Autodesk Fusion 360 part; units mm, degrees
(part 13 of 14)
  line L9122 (-513.1939, 44.45) -> (-524.1924, 44.45)
  line L9123 (-524.1924, 44.45) -> (-529.6916, 34.925)
  line L9124 (-529.6916, 34.925) -> (-524.1924, 25.4)
  line L9125 (-524.1924, 25.4) -> (-513.1939, 25.4)
  line L9126 (-507.6946, 34.925) -> (-513.1939, 44.45)
  line L9127 (-513.1939, 25.4) -> (-507.6946, 34.925)
  line L9128 (-493.9464, 55.5625) -> (-504.945, 55.5625)
  line L9129 (-504.945, 55.5625) -> (-510.4442, 46.0375)
  line L9130 (-510.4442, 46.0375) -> (-504.945, 36.5125)
  line L9131 (-504.945, 36.5125) -> (-493.9464, 36.5125)
  line L9132 (-488.4472, 46.0375) -> (-493.9464, 55.5625)
  line L9133 (-493.9464, 36.5125) -> (-488.4472, 46.0375)
  line L9134 (-474.699, 66.675) -> (-485.6976, 66.675)
  line L9135 (-485.6976, 66.675) -> (-491.1968, 57.15)
  line L9136 (-491.1968, 57.15) -> (-485.6976, 47.625)
  line L9137 (-485.6976, 47.625) -> (-474.699, 47.625)
  line L9138 (-469.1998, 57.15) -> (-474.699, 66.675)
  line L9139 (-474.699, 47.625) -> (-469.1998, 57.15)
  line L9140 (-455.4516, 77.7875) -> (-466.4501, 77.7875)
  line L9141 (-466.4501, 77.7875) -> (-471.9494, 68.2625)
  line L9142 (-471.9494, 68.2625) -> (-466.4501, 58.7375)
  line L9143 (-466.4501, 58.7375) -> (-455.4516, 58.7375)
  line L9144 (-449.9524, 68.2625) -> (-455.4516, 77.7875)
  line L9145 (-455.4516, 58.7375) -> (-449.9524, 68.2625)
  line L9146 (-436.2042, 88.9) -> (-447.2027, 88.9)
  line L9147 (-447.2027, 88.9) -> (-452.702, 79.375)
  line L9148 (-452.702, 79.375) -> (-447.2027, 69.85)
  line L9149 (-447.2027, 69.85) -> (-436.2042, 69.85)
  line L9150 (-430.7049, 79.375) -> (-436.2042, 88.9)
  line L9151 (-436.2042, 69.85) -> (-430.7049, 79.375)
  line L9152 (-416.9568, 100.0125) -> (-427.9553, 100.0125)
  line L9153 (-427.9553, 100.0125) -> (-433.4546, 90.4875)
  line L9154 (-433.4546, 90.4875) -> (-427.9553, 80.9625)
  line L9155 (-427.9553, 80.9625) -> (-416.9568, 80.9625)
  line L9156 (-411.4575, 90.4875) -> (-416.9568, 100.0125)
  line L9157 (-416.9568, 80.9625) -> (-411.4575, 90.4875)
  line L9158 (-397.7094, 111.125) -> (-408.7079, 111.125)
  line L9159 (-408.7079, 111.125) -> (-414.2072, 101.6)
  line L9160 (-414.2072, 101.6) -> (-408.7079, 92.075)
  line L9161 (-408.7079, 92.075) -> (-397.7094, 92.075)
  line L9162 (-392.2101, 101.6) -> (-397.7094, 111.125)
  line L9163 (-397.7094, 92.075) -> (-392.2101, 101.6)
  line L9164 (-378.462, 122.2375) -> (-389.4605, 122.2375)
  line L9165 (-389.4605, 122.2375) -> (-394.9597, 112.7125)
  line L9166 (-394.9597, 112.7125) -> (-389.4605, 103.1875)
  line L9167 (-389.4605, 103.1875) -> (-378.462, 103.1875)
  line L9168 (-372.9627, 112.7125) -> (-378.462, 122.2375)
  line L9169 (-378.462, 103.1875) -> (-372.9627, 112.7125)
  line L9170 (-359.2145, 133.35) -> (-370.2131, 133.35)
  line L9171 (-370.2131, 133.35) -> (-375.7123, 123.825)
  line L9172 (-375.7123, 123.825) -> (-370.2131, 114.3)
  line L9173 (-370.2131, 114.3) -> (-359.2145, 114.3)
  line L9174 (-353.7153, 123.825) -> (-359.2145, 133.35)
  line L9175 (-359.2145, 114.3) -> (-353.7153, 123.825)
  line L9176 (-339.9671, 144.4625) -> (-350.9657, 144.4625)
  line L9177 (-350.9657, 144.4625) -> (-356.4649, 134.9375)
  line L9178 (-356.4649, 134.9375) -> (-350.9657, 125.4125)
  line L9179 (-350.9657, 125.4125) -> (-339.9671, 125.4125)
  line L9180 (-334.4679, 134.9375) -> (-339.9671, 144.4625)
  line L9181 (-339.9671, 125.4125) -> (-334.4679, 134.9375)
  line L9182 (-320.7197, 155.575) -> (-331.7182, 155.575)
  line L9183 (-331.7182, 155.575) -> (-337.2175, 146.05)
  line L9184 (-337.2175, 146.05) -> (-331.7182, 136.525)
  line L9185 (-331.7182, 136.525) -> (-320.7197, 136.525)
  line L9186 (-315.2205, 146.05) -> (-320.7197, 155.575)
  line L9187 (-320.7197, 136.525) -> (-315.2205, 146.05)
  line L9188 (-301.4723, 166.6875) -> (-312.4708, 166.6875)
  line L9189 (-312.4708, 166.6875) -> (-317.9701, 157.1625)
  line L9190 (-317.9701, 157.1625) -> (-312.4708, 147.6375)
  line L9191 (-312.4708, 147.6375) -> (-301.4723, 147.6375)
  line L9192 (-295.973, 157.1625) -> (-301.4723, 166.6875)
  line L9193 (-301.4723, 147.6375) -> (-295.973, 157.1625)
  line L9194 (-282.2249, 177.8) -> (-293.2234, 177.8)
  line L9195 (-293.2234, 177.8) -> (-298.7227, 168.275)
  line L9196 (-298.7227, 168.275) -> (-293.2234, 158.75)
  line L9197 (-293.2234, 158.75) -> (-282.2249, 158.75)
  line L9198 (-276.7256, 168.275) -> (-282.2249, 177.8)
  line L9199 (-282.2249, 158.75) -> (-276.7256, 168.275)
  line L9200 (-262.9775, 188.9125) -> (-273.976, 188.9125)
  line L9201 (-273.976, 188.9125) -> (-279.4753, 179.3875)
  line L9202 (-279.4753, 179.3875) -> (-273.976, 169.8625)
  line L9203 (-273.976, 169.8625) -> (-262.9775, 169.8625)
  line L9204 (-257.4782, 179.3875) -> (-262.9775, 188.9125)
  line L9205 (-262.9775, 169.8625) -> (-257.4782, 179.3875)
  line L9206 (-243.7301, 200.025) -> (-254.7286, 200.025)
  line L9207 (-254.7286, 200.025) -> (-260.2278, 190.5)
  line L9208 (-260.2278, 190.5) -> (-254.7286, 180.975)
  line L9209 (-254.7286, 180.975) -> (-243.7301, 180.975)
  line L9210 (-238.2308, 190.5) -> (-243.7301, 200.025)
  line L9211 (-243.7301, 180.975) -> (-238.2308, 190.5)
  line L9212 (-224.4826, 211.1375) -> (-235.4812, 211.1375)
  line L9213 (-235.4812, 211.1375) -> (-240.9804, 201.6125)
  line L9214 (-240.9804, 201.6125) -> (-235.4812, 192.0875)
  line L9215 (-235.4812, 192.0875) -> (-224.4826, 192.0875)
  line L9216 (-218.9834, 201.6125) -> (-224.4826, 211.1375)
  line L9217 (-224.4826, 192.0875) -> (-218.9834, 201.6125)
  line L9218 (-205.2352, 222.25) -> (-216.2337, 222.25)
  line L9219 (-216.2337, 222.25) -> (-221.733, 212.725)
  line L9220 (-221.733, 212.725) -> (-216.2337, 203.2)
  line L9221 (-216.2337, 203.2) -> (-205.2352, 203.2)
  line L9222 (-199.736, 212.725) -> (-205.2352, 222.25)
  line L9223 (-205.2352, 203.2) -> (-199.736, 212.725)
  line L9224 (-185.9878, 233.3625) -> (-196.9863, 233.3625)
  line L9225 (-196.9863, 233.3625) -> (-202.4856, 223.8375)
  line L9226 (-202.4856, 223.8375) -> (-196.9863, 214.3125)
  line L9227 (-196.9863, 214.3125) -> (-185.9878, 214.3125)
  line L9228 (-180.4886, 223.8375) -> (-185.9878, 233.3625)
  line L9229 (-185.9878, 214.3125) -> (-180.4886, 223.8375)
  line L9230 (-166.7404, 244.475) -> (-177.7389, 244.475)
  line L9231 (-177.7389, 244.475) -> (-183.2382, 234.95)
  line L9232 (-183.2382, 234.95) -> (-177.7389, 225.425)
  line L9233 (-177.7389, 225.425) -> (-166.7404, 225.425)
  line L9234 (-161.2411, 234.95) -> (-166.7404, 244.475)
  line L9235 (-166.7404, 225.425) -> (-161.2411, 234.95)
  line L9236 (-147.493, 255.5875) -> (-158.4915, 255.5875)
  line L9237 (-158.4915, 255.5875) -> (-163.9908, 246.0625)
  line L9238 (-163.9908, 246.0625) -> (-158.4915, 236.5375)
  line L9239 (-158.4915, 236.5375) -> (-147.493, 236.5375)
  line L9240 (-141.9937, 246.0625) -> (-147.493, 255.5875)
  line L9241 (-147.493, 236.5375) -> (-141.9937, 246.0625)
  line L9242 (-128.2456, 266.7) -> (-139.2441, 266.7)
  line L9243 (-139.2441, 266.7) -> (-144.7434, 257.175)
  line L9244 (-144.7434, 257.175) -> (-139.2441, 247.65)
  line L9245 (-139.2441, 247.65) -> (-128.2456, 247.65)
  line L9246 (-122.7463, 257.175) -> (-128.2456, 266.7)
  line L9247 (-128.2456, 247.65) -> (-122.7463, 257.175)
  line L9248 (-108.9982, 277.8125) -> (-119.9967, 277.8125)
  line L9249 (-119.9967, 277.8125) -> (-125.4959, 268.2875)
  line L9250 (-125.4959, 268.2875) -> (-119.9967, 258.7625)
  line L9251 (-119.9967, 258.7625) -> (-108.9982, 258.7625)
  line L9252 (-103.4989, 268.2875) -> (-108.9982, 277.8125)
  line L9253 (-108.9982, 258.7625) -> (-103.4989, 268.2875)
  line L9254 (-89.7507, 288.925) -> (-100.7493, 288.925)
  line L9255 (-100.7493, 288.925) -> (-106.2485, 279.4)
  line L9256 (-106.2485, 279.4) -> (-100.7493, 269.875)
  line L9257 (-100.7493, 269.875) -> (-89.7507, 269.875)
  line L9258 (-84.2515, 279.4) -> (-89.7507, 288.925)
  line L9259 (-89.7507, 269.875) -> (-84.2515, 279.4)
  line L9260 (-70.5033, 300.0375) -> (-81.5018, 300.0375)
  line L9261 (-81.5018, 300.0375) -> (-87.0011, 290.5125)
  line L9262 (-87.0011, 290.5125) -> (-81.5018, 280.9875)
  line L9263 (-81.5018, 280.9875) -> (-70.5033, 280.9875)
  line L9264 (-65.0041, 290.5125) -> (-70.5033, 300.0375)
  line L9265 (-70.5033, 280.9875) -> (-65.0041, 290.5125)
  line L9266 (-51.2559, 311.15) -> (-62.2544, 311.15)
  line L9267 (-62.2544, 311.15) -> (-67.7537, 301.625)
  line L9268 (-67.7537, 301.625) -> (-62.2544, 292.1)
  line L9269 (-62.2544, 292.1) -> (-51.2559, 292.1)
  line L9270 (-45.7566, 301.625) -> (-51.2559, 311.15)
  line L9271 (-51.2559, 292.1) -> (-45.7566, 301.625)
  line L9272 (-32.0085, 322.2625) -> (-43.007, 322.2625)
  line L9273 (-43.007, 322.2625) -> (-48.5063, 312.7375)
  line L9274 (-48.5063, 312.7375) -> (-43.007, 303.2125)
  line L9275 (-43.007, 303.2125) -> (-32.0085, 303.2125)
  line L9276 (-26.5092, 312.7375) -> (-32.0085, 322.2625)
  line L9277 (-32.0085, 303.2125) -> (-26.5092, 312.7375)
  line L9278 (-12.7611, 333.375) -> (-23.7596, 333.375)
  line L9279 (-23.7596, 333.375) -> (-29.2589, 323.85)
  line L9280 (-29.2589, 323.85) -> (-23.7596, 314.325)
  line L9281 (-23.7596, 314.325) -> (-12.7611, 314.325)
  line L9282 (-7.2618, 323.85) -> (-12.7611, 333.375)
  line L9283 (-12.7611, 314.325) -> (-7.2618, 323.85)
  line L9284 (6.4863, 344.4875) -> (-4.5122, 344.4875)
  line L9285 (-4.5122, 344.4875) -> (-10.0114, 334.9625)
  line L9286 (-10.0114, 334.9625) -> (-4.5122, 325.4375)
  line L9287 (-4.5122, 325.4375) -> (6.4863, 325.4375)
  line L9288 (11.9856, 334.9625) -> (6.4863, 344.4875)
  line L9289 (6.4863, 325.4375) -> (11.9856, 334.9625)
  line L9290 (25.7337, 355.6) -> (14.7352, 355.6)
  line L9291 (14.7352, 355.6) -> (9.236, 346.075)
  line L9292 (9.236, 346.075) -> (14.7352, 336.55)
  line L9293 (14.7352, 336.55) -> (25.7337, 336.55)
  line L9294 (31.233, 346.075) -> (25.7337, 355.6)
  line L9295 (25.7337, 336.55) -> (31.233, 346.075)
  line L9296 (44.9812, 366.7125) -> (33.9826, 366.7125)
  line L9297 (33.9826, 366.7125) -> (28.4834, 357.1875)
  line L9298 (28.4834, 357.1875) -> (33.9826, 347.6625)
  line L9299 (33.9826, 347.6625) -> (44.9812, 347.6625)
  line L9300 (50.4804, 357.1875) -> (44.9812, 366.7125)
  line L9301 (44.9812, 347.6625) -> (50.4804, 357.1875)
  line L9302 (64.2286, 377.825) -> (53.2301, 377.825)
  line L9303 (53.2301, 377.825) -> (47.7308, 368.3)
  line L9304 (47.7308, 368.3) -> (53.2301, 358.775)
  line L9305 (53.2301, 358.775) -> (64.2286, 358.775)
  line L9306 (69.7278, 368.3) -> (64.2286, 377.825)
  line L9307 (64.2286, 358.775) -> (69.7278, 368.3)
  line L9308 (83.476, 388.9375) -> (72.4775, 388.9375)
  line L9309 (72.4775, 388.9375) -> (66.9782, 379.4125)
  line L9310 (66.9782, 379.4125) -> (72.4775, 369.8875)
  line L9311 (72.4775, 369.8875) -> (83.476, 369.8875)
  line L9312 (88.9753, 379.4125) -> (83.476, 388.9375)
  line L9313 (83.476, 369.8875) -> (88.9753, 379.4125)
  line L9314 (102.7234, 400.05) -> (91.7249, 400.05)
  line L9315 (91.7249, 400.05) -> (86.2256, 390.525)
  line L9316 (86.2256, 390.525) -> (91.7249, 381)
  line L9317 (91.7249, 381) -> (102.7234, 381)
  line L9318 (108.2227, 390.525) -> (102.7234, 400.05)
  line L9319 (102.7234, 381) -> (108.2227, 390.525)
  line L9320 (121.9708, 411.1625) -> (110.9723, 411.1625)
  line L9321 (110.9723, 411.1625) -> (105.473, 401.6375)
  line L9322 (105.473, 401.6375) -> (110.9723, 392.1125)
  line L9323 (110.9723, 392.1125) -> (121.9708, 392.1125)
  line L9324 (127.4701, 401.6375) -> (121.9708, 411.1625)
  line L9325 (121.9708, 392.1125) -> (127.4701, 401.6375)
  line L9326 (141.2182, 422.275) -> (130.2197, 422.275)
  line L9327 (130.2197, 422.275) -> (124.7205, 412.75)
  line L9328 (124.7205, 412.75) -> (130.2197, 403.225)
  line L9329 (130.2197, 403.225) -> (141.2182, 403.225)
  line L9330 (146.7175, 412.75) -> (141.2182, 422.275)
  line L9331 (141.2182, 403.225) -> (146.7175, 412.75)
  line L9332 (160.4657, 433.3875) -> (149.4671, 433.3875)
  line L9333 (149.4671, 433.3875) -> (143.9679, 423.8625)
  line L9334 (143.9679, 423.8625) -> (149.4671, 414.3375)
  line L9335 (149.4671, 414.3375) -> (160.4657, 414.3375)
  line L9336 (165.9649, 423.8625) -> (160.4657, 433.3875)
  line L9337 (160.4657, 414.3375) -> (165.9649, 423.8625)
  line L9338 (179.7131, 444.5) -> (168.7145, 444.5)
  line L9339 (168.7145, 444.5) -> (163.2153, 434.975)
  line L9340 (163.2153, 434.975) -> (168.7145, 425.45)
  line L9341 (168.7145, 425.45) -> (179.7131, 425.45)
  line L9342 (185.2123, 434.975) -> (179.7131, 444.5)
  line L9343 (179.7131, 425.45) -> (185.2123, 434.975)
  line L9344 (198.9605, 455.6125) -> (187.962, 455.6125)
  line L9345 (187.962, 455.6125) -> (182.4627, 446.0875)
  line L9346 (182.4627, 446.0875) -> (187.962, 436.5625)
  line L9347 (187.962, 436.5625) -> (198.9605, 436.5625)
  line L9348 (204.4597, 446.0875) -> (198.9605, 455.6125)
  line L9349 (198.9605, 436.5625) -> (204.4597, 446.0875)
  line L9350 (218.2079, 466.725) -> (207.2094, 466.725)
  line L9351 (207.2094, 466.725) -> (201.7101, 457.2)
  line L9352 (201.7101, 457.2) -> (207.2094, 447.675)
  line L9353 (207.2094, 447.675) -> (218.2079, 447.675)
  line L9354 (223.7072, 457.2) -> (218.2079, 466.725)
  line L9355 (218.2079, 447.675) -> (223.7072, 457.2)
  line L9356 (237.4553, 477.8375) -> (226.4568, 477.8375)
  line L9357 (226.4568, 477.8375) -> (220.9575, 468.3125)
  line L9358 (220.9575, 468.3125) -> (226.4568, 458.7875)
  line L9359 (226.4568, 458.7875) -> (237.4553, 458.7875)
  line L9360 (242.9546, 468.3125) -> (237.4553, 477.8375)
  line L9361 (237.4553, 458.7875) -> (242.9546, 468.3125)
  line L9362 (256.7027, 488.95) -> (245.7042, 488.95)
  line L9363 (245.7042, 488.95) -> (240.2049, 479.425)
  line L9364 (240.2049, 479.425) -> (245.7042, 469.9)
  line L9365 (245.7042, 469.9) -> (256.7027, 469.9)
  line L9366 (262.202, 479.425) -> (256.7027, 488.95)
  line L9367 (256.7027, 469.9) -> (262.202, 479.425)
  line L9368 (275.9501, 500.0625) -> (264.9516, 500.0625)
  line L9369 (264.9516, 500.0625) -> (259.4524, 490.5375)
  line L9370 (259.4524, 490.5375) -> (264.9516, 481.0125)
  line L9371 (264.9516, 481.0125) -> (275.9501, 481.0125)
  line L9372 (281.4494, 490.5375) -> (275.9501, 500.0625)
  line L9373 (275.9501, 481.0125) -> (281.4494, 490.5375)
  line L9374 (-878.8947, -144.4625) -> (-889.8933, -144.4625)
  line L9375 (-889.8933, -144.4625) -> (-895.3925, -153.9875)
  line L9376 (-895.3925, -153.9875) -> (-889.8933, -163.5125)
  line L9377 (-889.8933, -163.5125) -> (-878.8947, -163.5125)
  line L9378 (-873.3955, -153.9875) -> (-878.8947, -144.4625)
  line L9379 (-878.8947, -163.5125) -> (-873.3955, -153.9875)
  line L9380 (-859.6473, -133.35) -> (-870.6458, -133.35)
  line L9381 (-870.6458, -133.35) -> (-876.1451, -142.875)
  line L9382 (-876.1451, -142.875) -> (-870.6458, -152.4)
  line L9383 (-870.6458, -152.4) -> (-859.6473, -152.4)
  line L9384 (-854.1481, -142.875) -> (-859.6473, -133.35)
  line L9385 (-859.6473, -152.4) -> (-854.1481, -142.875)
  line L9386 (-840.3999, -122.2375) -> (-851.3984, -122.2375)
  line L9387 (-851.3984, -122.2375) -> (-856.8977, -131.7625)
  line L9388 (-856.8977, -131.7625) -> (-851.3984, -141.2875)
  line L9389 (-851.3984, -141.2875) -> (-840.3999, -141.2875)
  line L9390 (-834.9006, -131.7625) -> (-840.3999, -122.2375)
  line L9391 (-840.3999, -141.2875) -> (-834.9006, -131.7625)
  line L9392 (-821.1525, -111.125) -> (-832.151, -111.125)
  line L9393 (-832.151, -111.125) -> (-837.6503, -120.65)
  line L9394 (-837.6503, -120.65) -> (-832.151, -130.175)
  line L9395 (-832.151, -130.175) -> (-821.1525, -130.175)
  line L9396 (-815.6532, -120.65) -> (-821.1525, -111.125)
  line L9397 (-821.1525, -130.175) -> (-815.6532, -120.65)
  line L9398 (-801.9051, -100.0125) -> (-812.9036, -100.0125)
  line L9399 (-812.9036, -100.0125) -> (-818.4029, -109.5375)
  line L9400 (-818.4029, -109.5375) -> (-812.9036, -119.0625)
  line L9401 (-812.9036, -119.0625) -> (-801.9051, -119.0625)
  line L9402 (-796.4058, -109.5375) -> (-801.9051, -100.0125)
  line L9403 (-801.9051, -119.0625) -> (-796.4058, -109.5375)
  line L9404 (-782.6577, -88.9) -> (-793.6562, -88.9)
  line L9405 (-793.6562, -88.9) -> (-799.1554, -98.425)
  line L9406 (-799.1554, -98.425) -> (-793.6562, -107.95)
  line L9407 (-793.6562, -107.95) -> (-782.6577, -107.95)
  line L9408 (-777.1584, -98.425) -> (-782.6577, -88.9)
  line L9409 (-782.6577, -107.95) -> (-777.1584, -98.425)
  line L9410 (-763.4102, -77.7875) -> (-774.4088, -77.7875)
  line L9411 (-774.4088, -77.7875) -> (-779.908, -87.3125)
  line L9412 (-779.908, -87.3125) -> (-774.4088, -96.8375)
  line L9413 (-774.4088, -96.8375) -> (-763.4102, -96.8375)
  line L9414 (-757.911, -87.3125) -> (-763.4102, -77.7875)
  line L9415 (-763.4102, -96.8375) -> (-757.911, -87.3125)
  line L9416 (-744.1628, -66.675) -> (-755.1614, -66.675)
  line L9417 (-755.1614, -66.675) -> (-760.6606, -76.2)
  line L9418 (-760.6606, -76.2) -> (-755.1614, -85.725)
  line L9419 (-755.1614, -85.725) -> (-744.1628, -85.725)
  line L9420 (-738.6636, -76.2) -> (-744.1628, -66.675)
  line L9421 (-744.1628, -85.725) -> (-738.6636, -76.2)
  line L9422 (-724.9154, -55.5625) -> (-735.9139, -55.5625)
  line L9423 (-735.9139, -55.5625) -> (-741.4132, -65.0875)
  line L9424 (-741.4132, -65.0875) -> (-735.9139, -74.6125)
  line L9425 (-735.9139, -74.6125) -> (-724.9154, -74.6125)
  line L9426 (-719.4162, -65.0875) -> (-724.9154, -55.5625)
  line L9427 (-724.9154, -74.6125) -> (-719.4162, -65.0875)
  line L9428 (-705.668, -44.45) -> (-716.6665, -44.45)
  line L9429 (-716.6665, -44.45) -> (-722.1658, -53.975)
  line L9430 (-722.1658, -53.975) -> (-716.6665, -63.5)
  line L9431 (-716.6665, -63.5) -> (-705.668, -63.5)
  line L9432 (-700.1687, -53.975) -> (-705.668, -44.45)
  line L9433 (-705.668, -63.5) -> (-700.1687, -53.975)
  line L9434 (-686.4206, -33.3375) -> (-697.4191, -33.3375)
  line L9435 (-697.4191, -33.3375) -> (-702.9184, -42.8625)
  line L9436 (-702.9184, -42.8625) -> (-697.4191, -52.3875)
  line L9437 (-697.4191, -52.3875) -> (-686.4206, -52.3875)
  line L9438 (-680.9213, -42.8625) -> (-686.4206, -33.3375)
  line L9439 (-686.4206, -52.3875) -> (-680.9213, -42.8625)
  line L9440 (-667.1732, -22.225) -> (-678.1717, -22.225)
  line L9441 (-678.1717, -22.225) -> (-683.671, -31.75)
  line L9442 (-683.671, -31.75) -> (-678.1717, -41.275)
  line L9443 (-678.1717, -41.275) -> (-667.1732, -41.275)
  line L9444 (-661.6739, -31.75) -> (-667.1732, -22.225)
  line L9445 (-667.1732, -41.275) -> (-661.6739, -31.75)
  line L9446 (-647.9258, -11.1125) -> (-658.9243, -11.1125)
  line L9447 (-658.9243, -11.1125) -> (-664.4235, -20.6375)
  line L9448 (-664.4235, -20.6375) -> (-658.9243, -30.1625)
  line L9449 (-658.9243, -30.1625) -> (-647.9258, -30.1625)
  line L9450 (-642.4265, -20.6375) -> (-647.9258, -11.1125)
  line L9451 (-647.9258, -30.1625) -> (-642.4265, -20.6375)
  line L9452 (-628.6783, 0) -> (-639.6769, 0)
  line L9453 (-639.6769, 0) -> (-645.1761, -9.525)
  line L9454 (-645.1761, -9.525) -> (-639.6769, -19.05)
  line L9455 (-639.6769, -19.05) -> (-628.6783, -19.05)
  line L9456 (-623.1791, -9.525) -> (-628.6783, 0)
  line L9457 (-628.6783, -19.05) -> (-623.1791, -9.525)
  line L9458 (-609.4309, 11.1125) -> (-620.4295, 11.1125)
  line L9459 (-620.4295, 11.1125) -> (-625.9287, 1.5875)
  line L9460 (-625.9287, 1.5875) -> (-620.4295, -7.9375)
  line L9461 (-620.4295, -7.9375) -> (-609.4309, -7.9375)
  line L9462 (-603.9317, 1.5875) -> (-609.4309, 11.1125)
  line L9463 (-609.4309, -7.9375) -> (-603.9317, 1.5875)
  line L9464 (-590.1835, 22.225) -> (-601.182, 22.225)
  line L9465 (-601.182, 22.225) -> (-606.6813, 12.7)
  line L9466 (-606.6813, 12.7) -> (-601.182, 3.175)
  line L9467 (-601.182, 3.175) -> (-590.1835, 3.175)
  line L9468 (-584.6843, 12.7) -> (-590.1835, 22.225)
  line L9469 (-590.1835, 3.175) -> (-584.6843, 12.7)
  line L9470 (-570.9361, 33.3375) -> (-581.9346, 33.3375)
  line L9471 (-581.9346, 33.3375) -> (-587.4339, 23.8125)
  line L9472 (-587.4339, 23.8125) -> (-581.9346, 14.2875)
  line L9473 (-581.9346, 14.2875) -> (-570.9361, 14.2875)
  line L9474 (-565.4368, 23.8125) -> (-570.9361, 33.3375)
  line L9475 (-570.9361, 14.2875) -> (-565.4368, 23.8125)
  line L9476 (-551.6887, 44.45) -> (-562.6872, 44.45)
  line L9477 (-562.6872, 44.45) -> (-568.1865, 34.925)
  line L9478 (-568.1865, 34.925) -> (-562.6872, 25.4)
  line L9479 (-562.6872, 25.4) -> (-551.6887, 25.4)
  line L9480 (-546.1894, 34.925) -> (-551.6887, 44.45)
  line L9481 (-551.6887, 25.4) -> (-546.1894, 34.925)
  line L9482 (-532.4413, 55.5625) -> (-543.4398, 55.5625)
  line L9483 (-543.4398, 55.5625) -> (-548.9391, 46.0375)
  line L9484 (-548.9391, 46.0375) -> (-543.4398, 36.5125)
  line L9485 (-543.4398, 36.5125) -> (-532.4413, 36.5125)
  line L9486 (-526.942, 46.0375) -> (-532.4413, 55.5625)
  line L9487 (-532.4413, 36.5125) -> (-526.942, 46.0375)
  line L9488 (-513.1939, 66.675) -> (-524.1924, 66.675)
  line L9489 (-524.1924, 66.675) -> (-529.6916, 57.15)
  line L9490 (-529.6916, 57.15) -> (-524.1924, 47.625)
  line L9491 (-524.1924, 47.625) -> (-513.1939, 47.625)
  line L9492 (-507.6946, 57.15) -> (-513.1939, 66.675)
  line L9493 (-513.1939, 47.625) -> (-507.6946, 57.15)
  line L9494 (-493.9464, 77.7875) -> (-504.945, 77.7875)
  line L9495 (-504.945, 77.7875) -> (-510.4442, 68.2625)
  line L9496 (-510.4442, 68.2625) -> (-504.945, 58.7375)
  line L9497 (-504.945, 58.7375) -> (-493.9464, 58.7375)
  line L9498 (-488.4472, 68.2625) -> (-493.9464, 77.7875)
  line L9499 (-493.9464, 58.7375) -> (-488.4472, 68.2625)
  line L9500 (-474.699, 88.9) -> (-485.6976, 88.9)
  line L9501 (-485.6976, 88.9) -> (-491.1968, 79.375)
  line L9502 (-491.1968, 79.375) -> (-485.6976, 69.85)
  line L9503 (-485.6976, 69.85) -> (-474.699, 69.85)
  line L9504 (-469.1998, 79.375) -> (-474.699, 88.9)
  line L9505 (-474.699, 69.85) -> (-469.1998, 79.375)
  line L9506 (-455.4516, 100.0125) -> (-466.4501, 100.0125)
  line L9507 (-466.4501, 100.0125) -> (-471.9494, 90.4875)
  line L9508 (-471.9494, 90.4875) -> (-466.4501, 80.9625)
  line L9509 (-466.4501, 80.9625) -> (-455.4516, 80.9625)
  line L9510 (-449.9524, 90.4875) -> (-455.4516, 100.0125)
  line L9511 (-455.4516, 80.9625) -> (-449.9524, 90.4875)
  line L9512 (-436.2042, 111.125) -> (-447.2027, 111.125)
  line L9513 (-447.2027, 111.125) -> (-452.702, 101.6)
  line L9514 (-452.702, 101.6) -> (-447.2027, 92.075)
  line L9515 (-447.2027, 92.075) -> (-436.2042, 92.075)
  line L9516 (-430.7049, 101.6) -> (-436.2042, 111.125)
  line L9517 (-436.2042, 92.075) -> (-430.7049, 101.6)
  line L9518 (-416.9568, 122.2375) -> (-427.9553, 122.2375)
  line L9519 (-427.9553, 122.2375) -> (-433.4546, 112.7125)
  line L9520 (-433.4546, 112.7125) -> (-427.9553, 103.1875)
  line L9521 (-427.9553, 103.1875) -> (-416.9568, 103.1875)
  line L9522 (-411.4575, 112.7125) -> (-416.9568, 122.2375)
  line L9523 (-416.9568, 103.1875) -> (-411.4575, 112.7125)
  line L9524 (-397.7094, 133.35) -> (-408.7079, 133.35)
  line L9525 (-408.7079, 133.35) -> (-414.2072, 123.825)
  line L9526 (-414.2072, 123.825) -> (-408.7079, 114.3)
  line L9527 (-408.7079, 114.3) -> (-397.7094, 114.3)
  line L9528 (-392.2101, 123.825) -> (-397.7094, 133.35)
  line L9529 (-397.7094, 114.3) -> (-392.2101, 123.825)
  line L9530 (-378.462, 144.4625) -> (-389.4605, 144.4625)
  line L9531 (-389.4605, 144.4625) -> (-394.9597, 134.9375)
  line L9532 (-394.9597, 134.9375) -> (-389.4605, 125.4125)
  line L9533 (-389.4605, 125.4125) -> (-378.462, 125.4125)
  line L9534 (-372.9627, 134.9375) -> (-378.462, 144.4625)
  line L9535 (-378.462, 125.4125) -> (-372.9627, 134.9375)
  line L9536 (-359.2145, 155.575) -> (-370.2131, 155.575)
  line L9537 (-370.2131, 155.575) -> (-375.7123, 146.05)
  line L9538 (-375.7123, 146.05) -> (-370.2131, 136.525)
  line L9539 (-370.2131, 136.525) -> (-359.2145, 136.525)
  line L9540 (-353.7153, 146.05) -> (-359.2145, 155.575)
  line L9541 (-359.2145, 136.525) -> (-353.7153, 146.05)
  line L9542 (-339.9671, 166.6875) -> (-350.9657, 166.6875)
  line L9543 (-350.9657, 166.6875) -> (-356.4649, 157.1625)
  line L9544 (-356.4649, 157.1625) -> (-350.9657, 147.6375)
  line L9545 (-350.9657, 147.6375) -> (-339.9671, 147.6375)
  line L9546 (-334.4679, 157.1625) -> (-339.9671, 166.6875)
  line L9547 (-339.9671, 147.6375) -> (-334.4679, 157.1625)
  line L9548 (-320.7197, 177.8) -> (-331.7182, 177.8)
  line L9549 (-331.7182, 177.8) -> (-337.2175, 168.275)
  line L9550 (-337.2175, 168.275) -> (-331.7182, 158.75)
  line L9551 (-331.7182, 158.75) -> (-320.7197, 158.75)
  line L9552 (-315.2205, 168.275) -> (-320.7197, 177.8)
  line L9553 (-320.7197, 158.75) -> (-315.2205, 168.275)
  line L9554 (-301.4723, 188.9125) -> (-312.4708, 188.9125)
  line L9555 (-312.4708, 188.9125) -> (-317.9701, 179.3875)
  line L9556 (-317.9701, 179.3875) -> (-312.4708, 169.8625)
  line L9557 (-312.4708, 169.8625) -> (-301.4723, 169.8625)
  line L9558 (-295.973, 179.3875) -> (-301.4723, 188.9125)
  line L9559 (-301.4723, 169.8625) -> (-295.973, 179.3875)
  line L9560 (-282.2249, 200.025) -> (-293.2234, 200.025)
  line L9561 (-293.2234, 200.025) -> (-298.7227, 190.5)
  line L9562 (-298.7227, 190.5) -> (-293.2234, 180.975)
  line L9563 (-293.2234, 180.975) -> (-282.2249, 180.975)
  line L9564 (-276.7256, 190.5) -> (-282.2249, 200.025)
  line L9565 (-282.2249, 180.975) -> (-276.7256, 190.5)
  line L9566 (-262.9775, 211.1375) -> (-273.976, 211.1375)
  line L9567 (-273.976, 211.1375) -> (-279.4753, 201.6125)
  line L9568 (-279.4753, 201.6125) -> (-273.976, 192.0875)
  line L9569 (-273.976, 192.0875) -> (-262.9775, 192.0875)
  line L9570 (-257.4782, 201.6125) -> (-262.9775, 211.1375)
  line L9571 (-262.9775, 192.0875) -> (-257.4782, 201.6125)
  line L9572 (-243.7301, 222.25) -> (-254.7286, 222.25)
  line L9573 (-254.7286, 222.25) -> (-260.2278, 212.725)
  line L9574 (-260.2278, 212.725) -> (-254.7286, 203.2)
  line L9575 (-254.7286, 203.2) -> (-243.7301, 203.2)
  line L9576 (-238.2308, 212.725) -> (-243.7301, 222.25)
  line L9577 (-243.7301, 203.2) -> (-238.2308, 212.725)
  line L9578 (-224.4826, 233.3625) -> (-235.4812, 233.3625)
  line L9579 (-235.4812, 233.3625) -> (-240.9804, 223.8375)
  line L9580 (-240.9804, 223.8375) -> (-235.4812, 214.3125)
  line L9581 (-235.4812, 214.3125) -> (-224.4826, 214.3125)
  line L9582 (-218.9834, 223.8375) -> (-224.4826, 233.3625)
  line L9583 (-224.4826, 214.3125) -> (-218.9834, 223.8375)
  line L9584 (-205.2352, 244.475) -> (-216.2337, 244.475)
  line L9585 (-216.2337, 244.475) -> (-221.733, 234.95)
  line L9586 (-221.733, 234.95) -> (-216.2337, 225.425)
  line L9587 (-216.2337, 225.425) -> (-205.2352, 225.425)
  line L9588 (-199.736, 234.95) -> (-205.2352, 244.475)
  line L9589 (-205.2352, 225.425) -> (-199.736, 234.95)
  line L9590 (-185.9878, 255.5875) -> (-196.9863, 255.5875)
  line L9591 (-196.9863, 255.5875) -> (-202.4856, 246.0625)
  line L9592 (-202.4856, 246.0625) -> (-196.9863, 236.5375)
  line L9593 (-196.9863, 236.5375) -> (-185.9878, 236.5375)
  line L9594 (-180.4886, 246.0625) -> (-185.9878, 255.5875)
  line L9595 (-185.9878, 236.5375) -> (-180.4886, 246.0625)
  line L9596 (-166.7404, 266.7) -> (-177.7389, 266.7)
  line L9597 (-177.7389, 266.7) -> (-183.2382, 257.175)
  line L9598 (-183.2382, 257.175) -> (-177.7389, 247.65)
  line L9599 (-177.7389, 247.65) -> (-166.7404, 247.65)
  line L9600 (-161.2411, 257.175) -> (-166.7404, 266.7)
  line L9601 (-166.7404, 247.65) -> (-161.2411, 257.175)
  line L9602 (-147.493, 277.8125) -> (-158.4915, 277.8125)
  line L9603 (-158.4915, 277.8125) -> (-163.9908, 268.2875)
  line L9604 (-163.9908, 268.2875) -> (-158.4915, 258.7625)
  line L9605 (-158.4915, 258.7625) -> (-147.493, 258.7625)
  line L9606 (-141.9937, 268.2875) -> (-147.493, 277.8125)
  line L9607 (-147.493, 258.7625) -> (-141.9937, 268.2875)
  line L9608 (-128.2456, 288.925) -> (-139.2441, 288.925)
  line L9609 (-139.2441, 288.925) -> (-144.7434, 279.4)
  line L9610 (-144.7434, 279.4) -> (-139.2441, 269.875)
  line L9611 (-139.2441, 269.875) -> (-128.2456, 269.875)
  line L9612 (-122.7463, 279.4) -> (-128.2456, 288.925)
  line L9613 (-128.2456, 269.875) -> (-122.7463, 279.4)
  line L9614 (-108.9982, 300.0375) -> (-119.9967, 300.0375)
  line L9615 (-119.9967, 300.0375) -> (-125.4959, 290.5125)
  line L9616 (-125.4959, 290.5125) -> (-119.9967, 280.9875)
  line L9617 (-119.9967, 280.9875) -> (-108.9982, 280.9875)
  line L9618 (-103.4989, 290.5125) -> (-108.9982, 300.0375)
  line L9619 (-108.9982, 280.9875) -> (-103.4989, 290.5125)
  line L9620 (-89.7507, 311.15) -> (-100.7493, 311.15)
  line L9621 (-100.7493, 311.15) -> (-106.2485, 301.625)
  line L9622 (-106.2485, 301.625) -> (-100.7493, 292.1)
  line L9623 (-100.7493, 292.1) -> (-89.7507, 292.1)
  line L9624 (-84.2515, 301.625) -> (-89.7507, 311.15)
  line L9625 (-89.7507, 292.1) -> (-84.2515, 301.625)
  line L9626 (-70.5033, 322.2625) -> (-81.5018, 322.2625)
  line L9627 (-81.5018, 322.2625) -> (-87.0011, 312.7375)
  line L9628 (-87.0011, 312.7375) -> (-81.5018, 303.2125)
  line L9629 (-81.5018, 303.2125) -> (-70.5033, 303.2125)
  line L9630 (-65.0041, 312.7375) -> (-70.5033, 322.2625)
  line L9631 (-70.5033, 303.2125) -> (-65.0041, 312.7375)
  line L9632 (-51.2559, 333.375) -> (-62.2544, 333.375)
  line L9633 (-62.2544, 333.375) -> (-67.7537, 323.85)
  line L9634 (-67.7537, 323.85) -> (-62.2544, 314.325)
  line L9635 (-62.2544, 314.325) -> (-51.2559, 314.325)
  line L9636 (-45.7566, 323.85) -> (-51.2559, 333.375)
  line L9637 (-51.2559, 314.325) -> (-45.7566, 323.85)
  line L9638 (-32.0085, 344.4875) -> (-43.007, 344.4875)
  line L9639 (-43.007, 344.4875) -> (-48.5063, 334.9625)
  line L9640 (-48.5063, 334.9625) -> (-43.007, 325.4375)
  line L9641 (-43.007, 325.4375) -> (-32.0085, 325.4375)
  line L9642 (-26.5092, 334.9625) -> (-32.0085, 344.4875)
  line L9643 (-32.0085, 325.4375) -> (-26.5092, 334.9625)
  line L9644 (-12.7611, 355.6) -> (-23.7596, 355.6)
  line L9645 (-23.7596, 355.6) -> (-29.2589, 346.075)
  line L9646 (-29.2589, 346.075) -> (-23.7596, 336.55)
  line L9647 (-23.7596, 336.55) -> (-12.7611, 336.55)
  line L9648 (-7.2618, 346.075) -> (-12.7611, 355.6)
  line L9649 (-12.7611, 336.55) -> (-7.2618, 346.075)
  line L9650 (6.4863, 366.7125) -> (-4.5122, 366.7125)
  line L9651 (-4.5122, 366.7125) -> (-10.0114, 357.1875)
  line L9652 (-10.0114, 357.1875) -> (-4.5122, 347.6625)
  line L9653 (-4.5122, 347.6625) -> (6.4863, 347.6625)
  line L9654 (11.9856, 357.1875) -> (6.4863, 366.7125)
  line L9655 (6.4863, 347.6625) -> (11.9856, 357.1875)
  line L9656 (25.7337, 377.825) -> (14.7352, 377.825)
  line L9657 (14.7352, 377.825) -> (9.236, 368.3)
  line L9658 (9.236, 368.3) -> (14.7352, 358.775)
  line L9659 (14.7352, 358.775) -> (25.7337, 358.775)
  line L9660 (31.233, 368.3) -> (25.7337, 377.825)
  line L9661 (25.7337, 358.775) -> (31.233, 368.3)
  line L9662 (44.9812, 388.9375) -> (33.9826, 388.9375)
  line L9663 (33.9826, 388.9375) -> (28.4834, 379.4125)
  line L9664 (28.4834, 379.4125) -> (33.9826, 369.8875)
  line L9665 (33.9826, 369.8875) -> (44.9812, 369.8875)
  line L9666 (50.4804, 379.4125) -> (44.9812, 388.9375)
  line L9667 (44.9812, 369.8875) -> (50.4804, 379.4125)
  line L9668 (64.2286, 400.05) -> (53.2301, 400.05)
  line L9669 (53.2301, 400.05) -> (47.7308, 390.525)
  line L9670 (47.7308, 390.525) -> (53.2301, 381)
  line L9671 (53.2301, 381) -> (64.2286, 381)
  line L9672 (69.7278, 390.525) -> (64.2286, 400.05)
  line L9673 (64.2286, 381) -> (69.7278, 390.525)
  line L9674 (83.476, 411.1625) -> (72.4775, 411.1625)
  line L9675 (72.4775, 411.1625) -> (66.9782, 401.6375)
  line L9676 (66.9782, 401.6375) -> (72.4775, 392.1125)
  line L9677 (72.4775, 392.1125) -> (83.476, 392.1125)
  line L9678 (88.9753, 401.6375) -> (83.476, 411.1625)
  line L9679 (83.476, 392.1125) -> (88.9753, 401.6375)
  line L9680 (102.7234, 422.275) -> (91.7249, 422.275)
  line L9681 (91.7249, 422.275) -> (86.2256, 412.75)
  line L9682 (86.2256, 412.75) -> (91.7249, 403.225)
  line L9683 (91.7249, 403.225) -> (102.7234, 403.225)
  line L9684 (108.2227, 412.75) -> (102.7234, 422.275)
  line L9685 (102.7234, 403.225) -> (108.2227, 412.75)
  line L9686 (121.9708, 433.3875) -> (110.9723, 433.3875)
  line L9687 (110.9723, 433.3875) -> (105.473, 423.8625)
  line L9688 (105.473, 423.8625) -> (110.9723, 414.3375)
  line L9689 (110.9723, 414.3375) -> (121.9708, 414.3375)
  line L9690 (127.4701, 423.8625) -> (121.9708, 433.3875)
  line L9691 (121.9708, 414.3375) -> (127.4701, 423.8625)
  line L9692 (141.2182, 444.5) -> (130.2197, 444.5)
  line L9693 (130.2197, 444.5) -> (124.7205, 434.975)
  line L9694 (124.7205, 434.975) -> (130.2197, 425.45)
  line L9695 (130.2197, 425.45) -> (141.2182, 425.45)
  line L9696 (146.7175, 434.975) -> (141.2182, 444.5)
  line L9697 (141.2182, 425.45) -> (146.7175, 434.975)
  line L9698 (160.4657, 455.6125) -> (149.4671, 455.6125)
  line L9699 (149.4671, 455.6125) -> (143.9679, 446.0875)
  line L9700 (143.9679, 446.0875) -> (149.4671, 436.5625)
  line L9701 (149.4671, 436.5625) -> (160.4657, 436.5625)
  line L9702 (165.9649, 446.0875) -> (160.4657, 455.6125)
  line L9703 (160.4657, 436.5625) -> (165.9649, 446.0875)
  line L9704 (179.7131, 466.725) -> (168.7145, 466.725)
  line L9705 (168.7145, 466.725) -> (163.2153, 457.2)
  line L9706 (163.2153, 457.2) -> (168.7145, 447.675)
  line L9707 (168.7145, 447.675) -> (179.7131, 447.675)
  line L9708 (185.2123, 457.2) -> (179.7131, 466.725)
  line L9709 (179.7131, 447.675) -> (185.2123, 457.2)
  line L9710 (198.9605, 477.8375) -> (187.962, 477.8375)
  line L9711 (187.962, 477.8375) -> (182.4627, 468.3125)
  line L9712 (182.4627, 468.3125) -> (187.962, 458.7875)
  line L9713 (187.962, 458.7875) -> (198.9605, 458.7875)
  line L9714 (204.4597, 468.3125) -> (198.9605, 477.8375)
  line L9715 (198.9605, 458.7875) -> (204.4597, 468.3125)
  line L9716 (218.2079, 488.95) -> (207.2094, 488.95)
  line L9717 (207.2094, 488.95) -> (201.7101, 479.425)
  line L9718 (201.7101, 479.425) -> (207.2094, 469.9)
  line L9719 (207.2094, 469.9) -> (218.2079, 469.9)
  line L9720 (223.7072, 479.425) -> (218.2079, 488.95)
  line L9721 (218.2079, 469.9) -> (223.7072, 479.425)
  line L9722 (237.4553, 500.0625) -> (226.4568, 500.0625)
  line L9723 (226.4568, 500.0625) -> (220.9575, 490.5375)
  line L9724 (220.9575, 490.5375) -> (226.4568, 481.0125)
  line L9725 (226.4568, 481.0125) -> (237.4553, 481.0125)
  line L9726 (242.9546, 490.5375) -> (237.4553, 500.0625)
  line L9727 (237.4553, 481.0125) -> (242.9546, 490.5375)
  line L9728 (256.7027, 511.175) -> (245.7042, 511.175)
  line L9729 (245.7042, 511.175) -> (240.2049, 501.65)
  line L9730 (240.2049, 501.65) -> (245.7042, 492.125)
  line L9731 (245.7042, 492.125) -> (256.7027, 492.125)
  line L9732 (262.202, 501.65) -> (256.7027, 511.175)
  line L9733 (256.7027, 492.125) -> (262.202, 501.65)
  line L9734 (-898.1422, -133.35) -> (-909.1407, -133.35)
  line L9735 (-909.1407, -133.35) -> (-914.6399, -142.875)
  line L9736 (-914.6399, -142.875) -> (-909.1407, -152.4)
  line L9737 (-909.1407, -152.4) -> (-898.1422, -152.4)
  line L9738 (-892.6429, -142.875) -> (-898.1422, -133.35)
  line L9739 (-898.1422, -152.4) -> (-892.6429, -142.875)
  line L9740 (-878.8947, -122.2375) -> (-889.8933, -122.2375)
  line L9741 (-889.8933, -122.2375) -> (-895.3925, -131.7625)
  line L9742 (-895.3925, -131.7625) -> (-889.8933, -141.2875)
  line L9743 (-889.8933, -141.2875) -> (-878.8947, -141.2875)
  line L9744 (-873.3955, -131.7625) -> (-878.8947, -122.2375)
  line L9745 (-878.8947, -141.2875) -> (-873.3955, -131.7625)
  line L9746 (-859.6473, -111.125) -> (-870.6458, -111.125)
  line L9747 (-870.6458, -111.125) -> (-876.1451, -120.65)
  line L9748 (-876.1451, -120.65) -> (-870.6458, -130.175)
  line L9749 (-870.6458, -130.175) -> (-859.6473, -130.175)
  line L9750 (-854.1481, -120.65) -> (-859.6473, -111.125)
  line L9751 (-859.6473, -130.175) -> (-854.1481, -120.65)
  line L9752 (-840.3999, -100.0125) -> (-851.3984, -100.0125)
  line L9753 (-851.3984, -100.0125) -> (-856.8977, -109.5375)
  line L9754 (-856.8977, -109.5375) -> (-851.3984, -119.0625)
  line L9755 (-851.3984, -119.0625) -> (-840.3999, -119.0625)
  line L9756 (-834.9006, -109.5375) -> (-840.3999, -100.0125)
  line L9757 (-840.3999, -119.0625) -> (-834.9006, -109.5375)
  line L9758 (-821.1525, -88.9) -> (-832.151, -88.9)
  line L9759 (-832.151, -88.9) -> (-837.6503, -98.425)
  line L9760 (-837.6503, -98.425) -> (-832.151, -107.95)
  line L9761 (-832.151, -107.95) -> (-821.1525, -107.95)
  line L9762 (-815.6532, -98.425) -> (-821.1525, -88.9)
  line L9763 (-821.1525, -107.95) -> (-815.6532, -98.425)
  line L9764 (-801.9051, -77.7875) -> (-812.9036, -77.7875)
  line L9765 (-812.9036, -77.7875) -> (-818.4029, -87.3125)
  line L9766 (-818.4029, -87.3125) -> (-812.9036, -96.8375)
  line L9767 (-812.9036, -96.8375) -> (-801.9051, -96.8375)
  line L9768 (-796.4058, -87.3125) -> (-801.9051, -77.7875)
  line L9769 (-801.9051, -96.8375) -> (-796.4058, -87.3125)
  line L9770 (-782.6577, -66.675) -> (-793.6562, -66.675)
  line L9771 (-793.6562, -66.675) -> (-799.1554, -76.2)
  line L9772 (-799.1554, -76.2) -> (-793.6562, -85.725)
  line L9773 (-793.6562, -85.725) -> (-782.6577, -85.725)
  line L9774 (-777.1584, -76.2) -> (-782.6577, -66.675)
  line L9775 (-782.6577, -85.725) -> (-777.1584, -76.2)
  line L9776 (-763.4102, -55.5625) -> (-774.4088, -55.5625)
  line L9777 (-774.4088, -55.5625) -> (-779.908, -65.0875)
  line L9778 (-779.908, -65.0875) -> (-774.4088, -74.6125)
  line L9779 (-774.4088, -74.6125) -> (-763.4102, -74.6125)
  line L9780 (-757.911, -65.0875) -> (-763.4102, -55.5625)
  line L9781 (-763.4102, -74.6125) -> (-757.911, -65.0875)
  line L9782 (-744.1628, -44.45) -> (-755.1614, -44.45)
  line L9783 (-755.1614, -44.45) -> (-760.6606, -53.975)
  line L9784 (-760.6606, -53.975) -> (-755.1614, -63.5)
  line L9785 (-755.1614, -63.5) -> (-744.1628, -63.5)
  line L9786 (-738.6636, -53.975) -> (-744.1628, -44.45)
  line L9787 (-744.1628, -63.5) -> (-738.6636, -53.975)
  line L9788 (-724.9154, -33.3375) -> (-735.9139, -33.3375)
  line L9789 (-735.9139, -33.3375) -> (-741.4132, -42.8625)
  line L9790 (-741.4132, -42.8625) -> (-735.9139, -52.3875)
  line L9791 (-735.9139, -52.3875) -> (-724.9154, -52.3875)
  line L9792 (-719.4162, -42.8625) -> (-724.9154, -33.3375)
  line L9793 (-724.9154, -52.3875) -> (-719.4162, -42.8625)
  line L9794 (-705.668, -22.225) -> (-716.6665, -22.225)
  line L9795 (-716.6665, -22.225) -> (-722.1658, -31.75)
  line L9796 (-722.1658, -31.75) -> (-716.6665, -41.275)
  line L9797 (-716.6665, -41.275) -> (-705.668, -41.275)
  line L9798 (-700.1687, -31.75) -> (-705.668, -22.225)
  line L9799 (-705.668, -41.275) -> (-700.1687, -31.75)
  line L9800 (-686.4206, -11.1125) -> (-697.4191, -11.1125)
  line L9801 (-697.4191, -11.1125) -> (-702.9184, -20.6375)
  line L9802 (-702.9184, -20.6375) -> (-697.4191, -30.1625)
  line L9803 (-697.4191, -30.1625) -> (-686.4206, -30.1625)
  line L9804 (-680.9213, -20.6375) -> (-686.4206, -11.1125)
  line L9805 (-686.4206, -30.1625) -> (-680.9213, -20.6375)
  line L9806 (-667.1732, 0) -> (-678.1717, 0)
  line L9807 (-678.1717, 0) -> (-683.671, -9.525)
  line L9808 (-683.671, -9.525) -> (-678.1717, -19.05)
  line L9809 (-678.1717, -19.05) -> (-667.1732, -19.05)
  line L9810 (-661.6739, -9.525) -> (-667.1732, 0)
  line L9811 (-667.1732, -19.05) -> (-661.6739, -9.525)
  line L9812 (-647.9258, 11.1125) -> (-658.9243, 11.1125)
  line L9813 (-658.9243, 11.1125) -> (-664.4235, 1.5875)
  line L9814 (-664.4235, 1.5875) -> (-658.9243, -7.9375)
  line L9815 (-658.9243, -7.9375) -> (-647.9258, -7.9375)
  line L9816 (-642.4265, 1.5875) -> (-647.9258, 11.1125)
  line L9817 (-647.9258, -7.9375) -> (-642.4265, 1.5875)
  line L9818 (-628.6783, 22.225) -> (-639.6769, 22.225)
  line L9819 (-639.6769, 22.225) -> (-645.1761, 12.7)
  line L9820 (-645.1761, 12.7) -> (-639.6769, 3.175)
  line L9821 (-639.6769, 3.175) -> (-628.6783, 3.175)
  line L9822 (-623.1791, 12.7) -> (-628.6783, 22.225)
  line L9823 (-628.6783, 3.175) -> (-623.1791, 12.7)
  line L9824 (-609.4309, 33.3375) -> (-620.4295, 33.3375)
  line L9825 (-620.4295, 33.3375) -> (-625.9287, 23.8125)
  line L9826 (-625.9287, 23.8125) -> (-620.4295, 14.2875)
  line L9827 (-620.4295, 14.2875) -> (-609.4309, 14.2875)
  line L9828 (-603.9317, 23.8125) -> (-609.4309, 33.3375)
  line L9829 (-609.4309, 14.2875) -> (-603.9317, 23.8125)
  line L9830 (-590.1835, 44.45) -> (-601.182, 44.45)
  line L9831 (-601.182, 44.45) -> (-606.6813, 34.925)
  line L9832 (-606.6813, 34.925) -> (-601.182, 25.4)
  line L9833 (-601.182, 25.4) -> (-590.1835, 25.4)
  line L9834 (-584.6843, 34.925) -> (-590.1835, 44.45)
  line L9835 (-590.1835, 25.4) -> (-584.6843, 34.925)
  line L9836 (-570.9361, 55.5625) -> (-581.9346, 55.5625)
  line L9837 (-581.9346, 55.5625) -> (-587.4339, 46.0375)
  line L9838 (-587.4339, 46.0375) -> (-581.9346, 36.5125)
  line L9839 (-581.9346, 36.5125) -> (-570.9361, 36.5125)
  line L9840 (-565.4368, 46.0375) -> (-570.9361, 55.5625)
  line L9841 (-570.9361, 36.5125) -> (-565.4368, 46.0375)
  line L9842 (-551.6887, 66.675) -> (-562.6872, 66.675)
  line L9843 (-562.6872, 66.675) -> (-568.1865, 57.15)
  line L9844 (-568.1865, 57.15) -> (-562.6872, 47.625)
  line L9845 (-562.6872, 47.625) -> (-551.6887, 47.625)
  line L9846 (-546.1894, 57.15) -> (-551.6887, 66.675)
  line L9847 (-551.6887, 47.625) -> (-546.1894, 57.15)
  line L9848 (-532.4413, 77.7875) -> (-543.4398, 77.7875)
  line L9849 (-543.4398, 77.7875) -> (-548.9391, 68.2625)
  line L9850 (-548.9391, 68.2625) -> (-543.4398, 58.7375)
  line L9851 (-543.4398, 58.7375) -> (-532.4413, 58.7375)
  line L9852 (-526.942, 68.2625) -> (-532.4413, 77.7875)
  line L9853 (-532.4413, 58.7375) -> (-526.942, 68.2625)
  line L9854 (-513.1939, 88.9) -> (-524.1924, 88.9)
  line L9855 (-524.1924, 88.9) -> (-529.6916, 79.375)
  line L9856 (-529.6916, 79.375) -> (-524.1924, 69.85)
  line L9857 (-524.1924, 69.85) -> (-513.1939, 69.85)
  line L9858 (-507.6946, 79.375) -> (-513.1939, 88.9)
  line L9859 (-513.1939, 69.85) -> (-507.6946, 79.375)
  line L9860 (-493.9464, 100.0125) -> (-504.945, 100.0125)
  line L9861 (-504.945, 100.0125) -> (-510.4442, 90.4875)
  line L9862 (-510.4442, 90.4875) -> (-504.945, 80.9625)
  line L9863 (-504.945, 80.9625) -> (-493.9464, 80.9625)
  line L9864 (-488.4472, 90.4875) -> (-493.9464, 100.0125)
  line L9865 (-493.9464, 80.9625) -> (-488.4472, 90.4875)
  line L9866 (-474.699, 111.125) -> (-485.6976, 111.125)
  line L9867 (-485.6976, 111.125) -> (-491.1968, 101.6)
  line L9868 (-491.1968, 101.6) -> (-485.6976, 92.075)
  line L9869 (-485.6976, 92.075) -> (-474.699, 92.075)
  line L9870 (-469.1998, 101.6) -> (-474.699, 111.125)
  line L9871 (-474.699, 92.075) -> (-469.1998, 101.6)
  line L9872 (-455.4516, 122.2375) -> (-466.4501, 122.2375)
  line L9873 (-466.4501, 122.2375) -> (-471.9494, 112.7125)
  line L9874 (-471.9494, 112.7125) -> (-466.4501, 103.1875)
  line L9875 (-466.4501, 103.1875) -> (-455.4516, 103.1875)
  line L9876 (-449.9524, 112.7125) -> (-455.4516, 122.2375)
  line L9877 (-455.4516, 103.1875) -> (-449.9524, 112.7125)
  line L9878 (-436.2042, 133.35) -> (-447.2027, 133.35)
  line L9879 (-447.2027, 133.35) -> (-452.702, 123.825)
  line L9880 (-452.702, 123.825) -> (-447.2027, 114.3)
  line L9881 (-447.2027, 114.3) -> (-436.2042, 114.3)
  line L9882 (-430.7049, 123.825) -> (-436.2042, 133.35)
  line L9883 (-436.2042, 114.3) -> (-430.7049, 123.825)
  line L9884 (-416.9568, 144.4625) -> (-427.9553, 144.4625)
  line L9885 (-427.9553, 144.4625) -> (-433.4546, 134.9375)
  line L9886 (-433.4546, 134.9375) -> (-427.9553, 125.4125)
  line L9887 (-427.9553, 125.4125) -> (-416.9568, 125.4125)
  line L9888 (-411.4575, 134.9375) -> (-416.9568, 144.4625)
  line L9889 (-416.9568, 125.4125) -> (-411.4575, 134.9375)
  line L9890 (-397.7094, 155.575) -> (-408.7079, 155.575)
  line L9891 (-408.7079, 155.575) -> (-414.2072, 146.05)
  line L9892 (-414.2072, 146.05) -> (-408.7079, 136.525)
  line L9893 (-408.7079, 136.525) -> (-397.7094, 136.525)
  line L9894 (-392.2101, 146.05) -> (-397.7094, 155.575)
  line L9895 (-397.7094, 136.525) -> (-392.2101, 146.05)
  line L9896 (-378.462, 166.6875) -> (-389.4605, 166.6875)
  line L9897 (-389.4605, 166.6875) -> (-394.9597, 157.1625)
  line L9898 (-394.9597, 157.1625) -> (-389.4605, 147.6375)
  line L9899 (-389.4605, 147.6375) -> (-378.462, 147.6375)
  line L9900 (-372.9627, 157.1625) -> (-378.462, 166.6875)
  line L9901 (-378.462, 147.6375) -> (-372.9627, 157.1625)
  line L9902 (-359.2145, 177.8) -> (-370.2131, 177.8)
  line L9903 (-370.2131, 177.8) -> (-375.7123, 168.275)
  line L9904 (-375.7123, 168.275) -> (-370.2131, 158.75)
  line L9905 (-370.2131, 158.75) -> (-359.2145, 158.75)
  line L9906 (-353.7153, 168.275) -> (-359.2145, 177.8)
  line L9907 (-359.2145, 158.75) -> (-353.7153, 168.275)
  line L9908 (-339.9671, 188.9125) -> (-350.9657, 188.9125)
  line L9909 (-350.9657, 188.9125) -> (-356.4649, 179.3875)
  line L9910 (-356.4649, 179.3875) -> (-350.9657, 169.8625)
  line L9911 (-350.9657, 169.8625) -> (-339.9671, 169.8625)
  line L9912 (-334.4679, 179.3875) -> (-339.9671, 188.9125)
  line L9913 (-339.9671, 169.8625) -> (-334.4679, 179.3875)
  line L9914 (-320.7197, 200.025) -> (-331.7182, 200.025)
  line L9915 (-331.7182, 200.025) -> (-337.2175, 190.5)
  line L9916 (-337.2175, 190.5) -> (-331.7182, 180.975)
  line L9917 (-331.7182, 180.975) -> (-320.7197, 180.975)
  line L9918 (-315.2205, 190.5) -> (-320.7197, 200.025)
  line L9919 (-320.7197, 180.975) -> (-315.2205, 190.5)
  line L9920 (-301.4723, 211.1375) -> (-312.4708, 211.1375)
  line L9921 (-312.4708, 211.1375) -> (-317.9701, 201.6125)
  line L9922 (-317.9701, 201.6125) -> (-312.4708, 192.0875)
  line L9923 (-312.4708, 192.0875) -> (-301.4723, 192.0875)
  line L9924 (-295.973, 201.6125) -> (-301.4723, 211.1375)
  line L9925 (-301.4723, 192.0875) -> (-295.973, 201.6125)
  line L9926 (-282.2249, 222.25) -> (-293.2234, 222.25)
  line L9927 (-293.2234, 222.25) -> (-298.7227, 212.725)
  line L9928 (-298.7227, 212.725) -> (-293.2234, 203.2)
  line L9929 (-293.2234, 203.2) -> (-282.2249, 203.2)
  line L9930 (-276.7256, 212.725) -> (-282.2249, 222.25)
  line L9931 (-282.2249, 203.2) -> (-276.7256, 212.725)
  line L9932 (-262.9775, 233.3625) -> (-273.976, 233.3625)
  line L9933 (-273.976, 233.3625) -> (-279.4753, 223.8375)
  line L9934 (-279.4753, 223.8375) -> (-273.976, 214.3125)
  line L9935 (-273.976, 214.3125) -> (-262.9775, 214.3125)
  line L9936 (-257.4782, 223.8375) -> (-262.9775, 233.3625)
  line L9937 (-262.9775, 214.3125) -> (-257.4782, 223.8375)
  line L9938 (-243.7301, 244.475) -> (-254.7286, 244.475)
  line L9939 (-254.7286, 244.475) -> (-260.2278, 234.95)
  line L9940 (-260.2278, 234.95) -> (-254.7286, 225.425)
  line L9941 (-254.7286, 225.425) -> (-243.7301, 225.425)
  line L9942 (-238.2308, 234.95) -> (-243.7301, 244.475)
  line L9943 (-243.7301, 225.425) -> (-238.2308, 234.95)
  line L9944 (-224.4826, 255.5875) -> (-235.4812, 255.5875)
  line L9945 (-235.4812, 255.5875) -> (-240.9804, 246.0625)
  line L9946 (-240.9804, 246.0625) -> (-235.4812, 236.5375)
  line L9947 (-235.4812, 236.5375) -> (-224.4826, 236.5375)
  line L9948 (-218.9834, 246.0625) -> (-224.4826, 255.5875)
  line L9949 (-224.4826, 236.5375) -> (-218.9834, 246.0625)
  line L9950 (-205.2352, 266.7) -> (-216.2337, 266.7)
  line L9951 (-216.2337, 266.7) -> (-221.733, 257.175)
  line L9952 (-221.733, 257.175) -> (-216.2337, 247.65)
  line L9953 (-216.2337, 247.65) -> (-205.2352, 247.65)
  line L9954 (-199.736, 257.175) -> (-205.2352, 266.7)
  line L9955 (-205.2352, 247.65) -> (-199.736, 257.175)
  line L9956 (-185.9878, 277.8125) -> (-196.9863, 277.8125)
  line L9957 (-196.9863, 277.8125) -> (-202.4856, 268.2875)
  line L9958 (-202.4856, 268.2875) -> (-196.9863, 258.7625)
  line L9959 (-196.9863, 258.7625) -> (-185.9878, 258.7625)
  line L9960 (-180.4886, 268.2875) -> (-185.9878, 277.8125)
  line L9961 (-185.9878, 258.7625) -> (-180.4886, 268.2875)
  line L9962 (-166.7404, 288.925) -> (-177.7389, 288.925)
  line L9963 (-177.7389, 288.925) -> (-183.2382, 279.4)
  line L9964 (-183.2382, 279.4) -> (-177.7389, 269.875)
  line L9965 (-177.7389, 269.875) -> (-166.7404, 269.875)
  line L9966 (-161.2411, 279.4) -> (-166.7404, 288.925)
  line L9967 (-166.7404, 269.875) -> (-161.2411, 279.4)
  line L9968 (-147.493, 300.0375) -> (-158.4915, 300.0375)
  line L9969 (-158.4915, 300.0375) -> (-163.9908, 290.5125)
  line L9970 (-163.9908, 290.5125) -> (-158.4915, 280.9875)
  line L9971 (-158.4915, 280.9875) -> (-147.493, 280.9875)
  line L9972 (-141.9937, 290.5125) -> (-147.493, 300.0375)
  line L9973 (-147.493, 280.9875) -> (-141.9937, 290.5125)
  line L9974 (-128.2456, 311.15) -> (-139.2441, 311.15)
  line L9975 (-139.2441, 311.15) -> (-144.7434, 301.625)
  line L9976 (-144.7434, 301.625) -> (-139.2441, 292.1)
  line L9977 (-139.2441, 292.1) -> (-128.2456, 292.1)
  line L9978 (-122.7463, 301.625) -> (-128.2456, 311.15)
  line L9979 (-128.2456, 292.1) -> (-122.7463, 301.625)
  line L9980 (-108.9982, 322.2625) -> (-119.9967, 322.2625)
  line L9981 (-119.9967, 322.2625) -> (-125.4959, 312.7375)
  line L9982 (-125.4959, 312.7375) -> (-119.9967, 303.2125)
  line L9983 (-119.9967, 303.2125) -> (-108.9982, 303.2125)
  line L9984 (-103.4989, 312.7375) -> (-108.9982, 322.2625)
  line L9985 (-108.9982, 303.2125) -> (-103.4989, 312.7375)
  line L9986 (-89.7507, 333.375) -> (-100.7493, 333.375)
  line L9987 (-100.7493, 333.375) -> (-106.2485, 323.85)
  line L9988 (-106.2485, 323.85) -> (-100.7493, 314.325)
  line L9989 (-100.7493, 314.325) -> (-89.7507, 314.325)
  line L9990 (-84.2515, 323.85) -> (-89.7507, 333.375)
  line L9991 (-89.7507, 314.325) -> (-84.2515, 323.85)
  line L9992 (-70.5033, 344.4875) -> (-81.5018, 344.4875)
  line L9993 (-81.5018, 344.4875) -> (-87.0011, 334.9625)
  line L9994 (-87.0011, 334.9625) -> (-81.5018, 325.4375)
  line L9995 (-81.5018, 325.4375) -> (-70.5033, 325.4375)